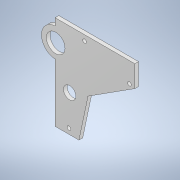
# Autodesk Inventor part: アームフレーム
Saved by Autodesk Inventor 2020.2 (Build 242310000, 310)
## iProperties
Created: 2020-02-29
Part Number: アームフレーム
Material: アルミニウム 2014-T4
Document SubType Name: Modeling
Designer: aoyam
Density: 2.8 g/cm^3
Appearance: サテン
Author: aoyam
Autodesk Inventor part; units mm, degrees
ref_plane "YZ Plane" through (0, 0, 0) normal (1, 0, 0) x (0, 1, 0)
ref_plane "XZ Plane" through (0, 0, 0) normal (0, 1, 0) x (-1, 0, 0)
ref_plane "XY Plane" through (0, 0, 0) normal (0, 0, 1) x (1, 0, 0)
sketch "ギア線図" plane through (0, 0, 0) normal (0, 0, 1) x (1, 0, 0)
  circle A0 centre (11.2246, -29.111) radius 11.1
  circle A1 centre (54.3074, -26.8895) radius 20.05
  circle A2 centre (54.3074, -26.8895) radius 4.55
  circle A3 centre (35.8191, -9.9133) radius 11.1
  circle A4 centre (39.3074, -43.38) radius 2.05
  circle A5 centre (69.3074, -43.38) radius 2.05
  circle A6 centre (72.141, -13.5141) radius 2.05
  circle A7 centre (39.3074, -43.38) radius 15
  circle A8 centre (69.3074, -43.38) radius 15
  circle A9 centre (72.141, -13.5141) radius 15
  circle A10 centre (54.3074, -26.8895) radius 5.5 construction
  circle A11 centre (11.2246, -29.111) radius 13 construction
  circle A12 centre (54.3074, -26.8895) radius 20.5 construction
  circle A13 centre (35.8191, -9.9133) radius 20.55
  circle A14 centre (35.8191, -9.9133) radius 21.5 construction
  circle A15 centre (35.8191, -9.9133) radius 13 construction
  circle A16 centre (39.3074, -43.38) radius 2.5 construction
  circle A17 centre (69.3074, -43.38) radius 2.5 construction
  circle A18 centre (72.141, -13.5141) radius 2.5 construction
  circle A19 centre (11.2246, -29.111) radius 20.1
  circle A20 centre (11.2246, -29.111) radius 22 construction
  line L0 (39.3074, -43.38) -> (69.3074, -43.38)
  circle A21 centre (0, 0) radius 20.1
  circle A22 centre (0, 0) radius 22 construction
  circle A23 centre (39.3074, -43.38) radius 9.5 construction
  circle A24 centre (69.3074, -43.38) radius 9.5 construction
  circle A25 centre (72.141, -13.5141) radius 9.5 construction
  point P0 (58.2233, -20.0465)
  point P1 (42.0436, -35)
  point P2 (21.5995, 15.2696)
  point P3 (38.2329, 5.9161)
  point P4 (24.1755, 8.4229)
  point P5 (21.6039, 15.1272)
  point P6 (23.3458, 16.3469)
  point P7 (23.3177, 16.3886)
  dimension "d7" = 22.2
  dimension "d8" = 40.1
  dimension "d9" = 9.1
  dimension "d11" = 22.2
  dimension "d12" = 4.1
  dimension "d13" = 4.1
  dimension "d14" = 4.1
  dimension "d15" = 30
  dimension "d16" = 30
  dimension "d17" = 30
  dimension "d18" = 11
  dimension "d21" = 26
  dimension "d29" = 41
  dimension "d39" = 22.2921
  dimension "d40" = 22.2921
  dimension "d41" = 22.2921
  dimension "d43" = 41.1
  dimension "d44" = 43
  dimension "d45" = 26
  dimension "d46" = 5
  dimension "d47" = 5
  dimension "d48" = 5
  dimension "d49" = 40.2
  dimension "d50" = 44
  dimension "d53" = 40.2
  dimension "d55" = 44
  dimension "d58" = 19
  dimension "d59" = 19
  dimension "d60" = 19
  constraints: 26 centre point, 15 coincident, 7 tangent, 3 concentric, 2 end point, 1 horizontal, 1 other
  measures "d7" diameter of A0
  measures "d8" diameter of A1
  measures "d9" diameter of A2
  measures "d11" diameter of A3
  measures "d12" diameter of A4
  measures "d13" diameter of A5
  measures "d14" diameter of A6
  measures "d15" diameter of A7
  measures "d16" diameter of A8
  measures "d17" diameter of A9
  measures "d18" diameter of A10
  measures "d21" diameter of A11
  measures "d29" diameter of A12
  measures "d39" distance of A4.centre A1.centre
  measures "d40" distance of A5.centre A1.centre
  measures "d41" distance of A6.centre A1.centre
  measures "d43" diameter of A13
  measures "d44" diameter of A14
  measures "d45" diameter of A15
  measures "d46" diameter of A16
  measures "d47" diameter of A17
  measures "d48" diameter of A18
  measures "d49" diameter of A19
  measures "d50" diameter of A20
  measures "d53" diameter of A21
  measures "d55" diameter of A22
  measures "d58" diameter of A23
  measures "d59" diameter of A24
  measures "d60" diameter of A25
sketch "スケッチ3" plane through (0, 0, 0) normal (0, 0, 1) x (1, 0, 0)
  circle A0 centre (11.2246, -29.111) radius 20.1 construction
  circle A1 centre (39.3074, -43.38) radius 15 construction
  circle A2 centre (69.3074, -43.38) radius 15 construction
  circle A3 centre (72.141, -13.5141) radius 15 construction
  circle A4 centre (11.2246, -29.111) radius 5
  circle A5 centre (59.3303, 1.1874) radius 1.5
  circle A6 centre (23.1948, 12.8161) radius 1.5
  circle A7 centre (10.6068, -54.0855) radius 1.5
  circle A8 centre (59.3303, 1.1874) radius 4.5 construction
  circle A9 centre (35.8191, -9.9133) radius 21.5 construction
  circle A10 centre (23.1948, 12.8161) radius 4.5 construction
  circle A11 centre (0, 0) radius 22 construction
  line L0 (18.6948, -58.38) -> (25.9736, -24.111)
  line L1 (25.9736, -24.111) -> (63.6708, 0)
  line L2 (63.6708, 17.3161) -> (-0.523, 17.3161)
  line L3 (-0.523, 17.3161) -> (-0.523, -58.38)
  line L4 (-0.523, -58.38) -> (18.6948, -58.38)
  line L5 (63.6708, 17.3161) -> (63.6708, 0)
  circle A12 centre (0, 0) radius 7.5
  circle A13 centre (0, 0) radius 11.5
  point P0 (-0.523, -11.4881)
  point P1 (-0.523, 11.4881)
  dimension "d69" = 9
  dimension "d61" = 10
  dimension "d63" = 3
  dimension "d64" = 3
  dimension "d67" = 3
  dimension "d70" = 9
  dimension "d71" = 15
  dimension "d72" = 4
  constraints: 12 end point, 7 centre point, 4 coincident, 2 perpendicular, 2 tangent, 1 horizontal, 5 other
  measures "d61" diameter of A4
  measures "d63" diameter of A5
  measures "d64" diameter of A6
  measures "d67" diameter of A7
  measures "d70" diameter of A10
  measures "d71" diameter of A12
  measures "d72" radial gap between concentric circles of A12 A13
extrude "押し出し1" add sketch "スケッチ3" along normal blind 3 contours L4 L3 A13 L2 L5 L1 L0 | A13 L3 A12 | L3 A12 A13
sketch "スケッチ4" plane through (0, 0, 3) normal (0, 0, 1) x (1, 0, 0)
  circle A0 centre (23.1948, 12.8161) radius 1.5 projected
  circle A1 centre (59.3303, 1.1874) radius 1.5 projected
  circle A2 centre (11.2246, -29.111) radius 5 projected
  circle A3 centre (10.6068, -54.0855) radius 1.5 projected
  point P0 (0, 0)
equation "\"d40\" = d39"
equation "\"d41\" = d40"
